# Autodesk Inventor part: arm
Saved by Autodesk Inventor 2021 (Build 250183000, 183)
## iProperties
Created: 2020-12-29
Part Number: arm
Material: ABS Plastic
Document SubType Name: Modeling
Designer: Tomasz
Density: 1.06 g/cm^3
Appearance: Smooth - Black
Author: Tomasz
Autodesk Inventor part; units mm, degrees
ref_plane "YZ Plane" through (0, 0, 0) normal (1, 0, 0) x (0, 1, 0)
ref_plane "XZ Plane" through (0, 0, 0) normal (0, 1, 0) x (-1, 0, 0)
ref_plane "XY Plane" through (0, 0, 0) normal (0, 0, 1) x (1, 0, 0)
sketch "arm_sketch" plane through (0, 0, 0) normal (0, 1, 0) x (-1, 0, 0)
  line L0 (0, -40) -> (-20, -40) construction
  line L1 (-20, -40) -> (-20, 0) construction
  line L2 (-20, 0) -> (0, 0) construction
  line L3 (0, 0) -> (0, -40) construction
  line L4 (0, -30) -> (-20, -30) construction
  line L5 (-20, -30) -> (-20, -10)
  line L6 (-20, -10) -> (0, -10) construction
  line L7 (0, -10) -> (0, -30) construction
  line L8 (-20, -40) -> (-34, -40)
  line L9 (-34, -40) -> (-34, -30)
  line L10 (-34, -30) -> (-20, -30)
  line L11 (-20, -30) -> (-20, -40) construction
  line L12 (0, -20) -> (-20, -20) construction
  line L13 (-10, -40) -> (-10, 0) construction
  line L14 (-20, 0) -> (-34, 0)
  line L15 (-34, 0) -> (-34, -10)
  line L16 (-34, -10) -> (-20, -10)
  line L17 (-20, -10) -> (-20, 0) construction
  line L18 (0, -40) -> (14, -40) construction
  line L19 (14, -40) -> (14, -30) construction
  line L20 (14, -30) -> (0, -30)
  line L21 (0, -30) -> (0, -40) construction
  line L22 (0, -10) -> (0, 0) construction
  line L23 (0, 0) -> (14, 0) construction
  line L24 (14, 0) -> (14, -10) construction
  line L25 (14, -10) -> (0, -10)
  line L26 (14, -30) -> (14, -10)
  line L27 (0, -10) -> (-8, -10)
  line L28 (-8, -10) -> (-8, 0)
  line L29 (0, -30) -> (-8, -30)
  line L30 (-8, -30) -> (-8, -40)
  line L31 (-8, -40) -> (-20, -40)
  line L32 (-8, 0) -> (-20, 0)
  point P0 (0, -10)
  point P1 (0, -10)
  dimension "d0" = 20
  dimension "d1" = 40
  dimension "d2" = 20
  dimension "d3" = 10
  dimension "d4" = 14
  dimension "d63" = 12
  dimension "d64" = 12
  constraints: 66 end point, 13 symmetric about line, 6 parallel, 6 point on line, 5 perpendicular, 4 midpoint, 3 horizontal, 2 coincident, 2 collinear, 1 vertical
  measures "d0" distance of L1.end L2.end
  measures "d1" distance of L0.end L1.end
  measures "d2" distance between parallel lines of L6 L4
  measures "d3" distance between parallel lines of L6 L2
  measures "d4" distance of L9.end L10.end
  measures "d63" distance between parallel lines of L1 L28
  measures "d64" distance between parallel lines of L1 L30
extrude "arm" add sketch "arm_sketch" along normal blind 10
sketch "Sketch5" plane through (8, 0, 0) normal (0, 0, 1) x (1, 0, 0)
  line L0 (26, 0) -> (26, 10) construction
  line L1 (26, 10) -> (12, 10) construction
  line L2 (-22, 0) -> (-22, 10) construction
  circle A0 centre (21, 5) radius 2
  circle A1 centre (-17, 5) radius 2
  dimension "d66" = 10
  dimension "d67" = 14
  dimension "d68" = 4
  dimension "d69" = 4
  dimension "d70" = 5
  dimension "d71" = 5
  dimension "d72" = 5
  dimension "d73" = 5
  constraints: 2 centre point
  measures "d66" distance of L0.start L0.end
  measures "d67" distance of L0.end L1.end
  measures "d68" diameter of A0
  measures "d69" diameter of A1
  measures "d70" distance from line of L2 A1.centre
  measures "d71" distance from line of A0.centre L0
  measures "d72" horizontal distance of L0.end A0.centre
  measures "d73" horizontal distance of L2.end A1.centre
extrude "rod_hole" cut sketch "Sketch5" against normal through all
fillet "rot_round" radius 4 12 edges at (-14, 10, -20) (-14, 0, -20) (34, 10, -35) (34, 0, -35) (34, 10, -5) (34, 0, -5) (8, 10, -5) (8, 0, -5) (8, 0, -35) (8, 10, -35) (20, 10, -20) (20, 0, -20)
equation "\"d3\" = 0.5 * d1 - 0.5 * d2"
equation "\"d64\" = d63"
equation "\"d68\" = arm_rod_diam"
equation "\"d69\" = arm_rod_diam"
equation "\"d70\" = d71"
equation "\"d71\" = d72"
equation "\"d72\" = 0.5 * d66"
equation "\"d73\" = d72"
equation "\"d76\" = arm_rod_diam"
equation "\"arm_rod_diam\" = 4"
equation "\"hole\" = 2.2"
body "Solid1"
